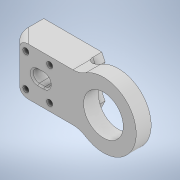
# Autodesk Inventor part: armtip_3
Saved by Autodesk Inventor 2020 (Build 240168000, 168)
## iProperties
Created: 2019-10-15
Part Number: armtip_3
Material: Generic
Document SubType Name: Modeling
Designer: psrob
Density: 1 g/cm^3
Appearance: Default
Author: psrob
Autodesk Inventor part; units mm, degrees
ref_plane "YZ Plane" through (0, 0, 0) normal (1, 0, 0) x (0, 1, 0)
ref_plane "XZ Plane" through (0, 0, 0) normal (0, 1, 0) x (-1, 0, 0)
ref_plane "XY Plane" through (0, 0, 0) normal (0, 0, 1) x (1, 0, 0)
sketch "Sketch1" plane through (0, 0, 0) normal (0, 0, 1) x (1, 0, 0)
  circle A0 centre (0, 0) radius 11 projected
  circle A1 centre (0, 0) radius 5 projected
  circle A2 centre (0, 0) radius 5.5
  circle A3 centre (0, 0) radius 11
  point P0 (0, 0)
  dimension "d0" = 11
  dimension "d1" = 22
  constraints: 2 centre point, 2 coincident
  measures "d0" diameter of A2
  measures "d1" diameter of A3
extrude "Extrusion1" add sketch "Sketch1" along normal blind 8 contours A0
sketch "Sketch3" plane through (0, 0, 8) normal (0, 0, 1) x (1, 0, 0)
  circle A0 centre (0, 0) radius 11 projected
  circle A1 centre (0, 0) radius 5.5 projected
  line L0 (0, 0) -> (-30, 0)
  line L1 (-30, 0) -> (-15, 0)
  line L2 (-30, 0) -> (-30, 8)
  line L3 (-30, 0) -> (-30, -8)
  line L4 (-30, -8) -> (-7.5498, -8)
  circle A2 centre (0, 0) radius 11 projected
  line L5 (-30, 8) -> (-7.5498, 8)
  point P0 (0, 0)
  point P1 (-7.5498, -8)
  dimension "d12" = 30
  dimension "d13" = 15
  dimension "d14" = 8
  dimension "d15" = 8
  constraints: 12 end point, 2 perpendicular, 2 point on circle, 1 horizontal, 1 midpoint, 1 parallel, 1 vertical
  measures "d12" distance of L0.start L0.end
  measures "d13" distance of L0.end L1.end
  measures "d14" distance of L0.end L2.end
  measures "d15" distance of L0.end L3.end
extrude "Extrusion3" add sketch "Sketch3" against normal blind 10 contours A0 L0 L2 L5 | L4 L3 L0 A0
sketch "Sketch4" plane through (0, 0, -2) normal (0, 0, -1) x (-1, 0, 0)
  line L0 (7.5498, -8) -> (30, -8) projected
  line L1 (30, -8) -> (30, 8) projected
  line L2 (30, 8) -> (7.5498, 8) projected
  line L3 (15, -3) -> (15, 3)
  line L4 (15, 3) -> (45, 3)
  line L5 (45, 3) -> (45, -3)
  line L6 (45, -3) -> (15, -3)
  line L7 (15, -3) -> (45, 3) construction
  line L8 (15, 3) -> (45, -3) construction
  line L9 (30, -8) -> (30, 8) projected
  arc A0 (7.5498, -8) -> (7.5498, 8) centre (0, 0) ccw projected
  point P0 (0, 0)
  point P1 (30, 0)
  point P2 (30, -3)
  point P3 (30, 3)
  dimension "d21" = 6
  dimension "d22" = 30
  constraints: 12 end point, 3 midpoint, 2 parallel, 2 perpendicular
  measures "d21" distance of L3.start L3.end
  measures "d22" distance of L3.end L4.end
extrude "Extrusion4" cut sketch "Sketch4" against normal blind 3 contours L6 L3 L4 L1
sketch "Sketch5" plane through (0, 0, -2) normal (0, 0, -1) x (-1, 0, 0)
  line L0 (15, 3) -> (30, 3) projected
  line L1 (30, 3) -> (30, 8) projected
  line L2 (30, 8) -> (7.5498, 8) projected
  line L3 (7.5498, -8) -> (30, -8) projected
  line L4 (30, -8) -> (30, -3) projected
  line L5 (30, -3) -> (15, -3) projected
  line L6 (15, -3) -> (15, 3) projected
  line L7 (30, 3) -> (30, -3) projected
  line L8 (30, 0) -> (26, 0)
  line L9 (26, 0) -> (26, -5.5)
  circle A0 centre (26, -5.5) radius 1
  line L10 (26, 0) -> (26, 5.5)
  circle A1 centre (26, 5.5) radius 1
  line L11 (26, -5.5) -> (18, -5.5)
  line L12 (18, -5.5) -> (18, 5.5)
  line L13 (18, 5.5) -> (26, 5.5)
  line L14 (26, 5.5) -> (26, -5.5)
  circle A2 centre (18, -5.5) radius 1
  circle A3 centre (18, 5.5) radius 1
  arc A4 (7.5498, -8) -> (7.5498, 8) centre (0, 0) ccw projected
  point P0 (0, 0)
  dimension "d25" = 4
  dimension "d26" = 5.5
  dimension "d27" = 2
  dimension "d28" = 5.5
  dimension "d29" = 2
  dimension "d30" = 8
  dimension "d31" = 11
  dimension "d32" = 2
  dimension "d33" = 2
  constraints: 14 end point, 4 centre point, 4 coincident, 2 horizontal, 2 parallel, 2 perpendicular, 1 midpoint, 1 vertical
  measures "d25" distance of L8.start L8.end
  measures "d26" distance of L8.end L9.end
  measures "d27" diameter of A0
  measures "d28" distance of L8.end L10.end
  measures "d29" diameter of A1
  measures "d30" distance of L12.end L13.end
  measures "d31" distance of L11.end L12.end
  measures "d32" diameter of A2
  measures "d33" diameter of A3
extrude "Extrusion5" cut sketch "Sketch5" against normal blind 10 contours A3 L13 L12 | L12 L13 A3 | A1 L13 L10 | L10 L13 A1 | A2 L11 L12 | L12 L11 A2 | A0 L11 L9 | L9 L11 A0
chamfer "Chamfer2" distance 2 angle 45 1 edges at (-30, 0, 8)
fillet "Fillet2" radius 2 2 edges at (-29, 8, 7) (-29, -8, 7)
thicken "Thicken1" operation add thickness 3 both sides no extend neighbours yes toward (0, 0, 1) faces at (-5.3528, -7.3729, 0)
sketch "Sketch6" plane through (0, 0, 3) normal (0, 0, -1) x (-1, 0, 0)
  arc A0 (7.5498, 8) -> (7.5498, -8) centre (0, 0) ccw projected
  arc A1 (7.5498, -8) -> (7.5498, 8) centre (0, 0) ccw projected
  circle A2 centre (0, 0) radius 5.5 projected
  circle A3 centre (0, 0) radius 6.5
  point P0 (0, 0)
  dimension "d43" = 13
  constraints: 1 centre point, 1 coincident
  measures "d43" diameter of A3
extrude "Extrusion6" cut sketch "Sketch6" against normal blind 10 contours A3
chamfer "Chamfer3" distance 3 angle 45 2 edges at (-7.5498, 8, 0.5) (-7.5498, -8, 0.5)
fillet "Fillet3" radius 2 3 edges at (-11, 0, 3) (-9.9902, 6.8313, 3) (-9.9902, -6.8313, 3)
fillet "Fillet4" radius 8 2 edges at (-7.5498, 8, 5.5) (-7.5498, -8, 5.5)
sketch "Sketch7" plane through (0, 0, 8) normal (0, 0, 1) x (1, 0, 0)
  circle A0 centre (0, 0) radius 6.5 projected
  ellipse E0 centre (-25.1716, -6) end of major axis (-28, -6) minor radius 2 (-28, -6) -> (-25.1716, -8) ccw projected
  line L0 (-25.1716, -8) -> (-10.247, -8) projected
  arc A1 (-5.9324, -9.2632) -> (-10.247, -8) centre (-10.247, -16) ccw projected
  arc A2 (-5.9324, -9.2632) -> (-5.9324, 9.2632) centre (0, 0) ccw projected
  arc A3 (-10.247, 8) -> (-5.9324, 9.2632) centre (-10.247, 16) ccw projected
  line L1 (-10.247, 8) -> (-25.1716, 8) projected
  ellipse E1 centre (-25.1716, 6) end of major axis (-28, 6) minor radius 2 (-25.1716, 8) -> (-28, 6) ccw projected
  line L2 (-28, -6) -> (-28, 6) projected
  circle A4 centre (-18, 5.5) radius 1 projected
  circle A5 centre (-26, 5.5) radius 1 projected
  circle A6 centre (-18, -5.5) radius 1 projected
  circle A7 centre (-26, -5.5) radius 1 projected
  circle A8 centre (-18, 5.5) radius 1 projected
  line L3 (-18, 5.5) -> (-18, -5.5)
  line L4 (-14, 0) -> (-22, 0) construction
  line L5 (-14, 2) -> (-22, 2)
  line L6 (-22, -2) -> (-14, -2)
  arc A9 (-14, -2) -> (-14, 2) centre (-14, 0) ccw
  arc A10 (-22, 2) -> (-22, -2) centre (-22, 0) ccw
  point P0 (0, 0)
  point P1 (-18, 0)
  point P2 (-18, -2)
  point P3 (-18, 2)
  dimension "d51" = 4
  dimension "d52" = 4
  constraints: 10 end point, 4 point on circle, 4 tangent, 2 centre point, 2 midpoint, 1 parallel, 1 perpendicular, 1 vertical, 2 other
  measures "d51" distance of point (-18, 0) L4.end
  measures "d52" diameter of A10
extrude "Extrusion7" cut sketch "Sketch7" against normal blind 10 contours L3 L6 A10 L5
fillet "Fillet5" radius 2 2 edges at (-18, -2, 4.5) (-18, 2, 4.5)
chamfer "Chamfer4" distance 0.5 angle 45 6 edges at (-18.5858, -1.4142, 8) (-18, 0, 8) (-18.5858, 1.4142, 8) (-20.9999, 2, 8) (-24, 0, 8) (-20.9999, -2, 8)
thicken "Thicken2" operation add thickness 0.15 both sides no extend neighbours yes toward (-0.9870503, -0.1604113, 0) faces at (-6.4158, -1.0427, 6.3333)
thicken "Thicken3" operation add thickness 0.1 both sides no extend neighbours yes toward (0, 1, 0) faces at (-25, 3, -1)
thicken "Thicken4" operation add thickness 0.1 both sides no extend neighbours yes toward (0, -1, 0) faces at (-20, -3, 0)
body "Solid1"
